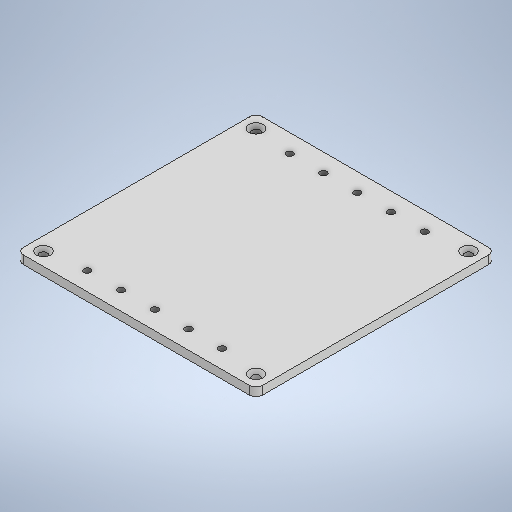
# Autodesk Inventor part: Chuck Adapter Plate
Saved by Autodesk Inventor 2025 (Build 290162000, 162)
## iProperties
Created: 2024-10-23
Part Number: Chuck Adapter Plate
Material: Generic
Document SubType Name: Modeling
Designer: Caleb Fangmeier
Density: 1 g/cm^3
Appearance: Default
Author: Caleb Fangmeier
Autodesk Inventor part; units mm, degrees
ref_plane "YZ Plane" through (0, 0, 0) normal (1, 0, 0) x (0, 1, 0)
ref_plane "XZ Plane" through (0, 0, 0) normal (0, 1, 0) x (-1, 0, 0)
ref_plane "XY Plane" through (0, 0, 0) normal (0, 0, 1) x (1, 0, 0)
sketch "Sketch1" plane through (0, 0, 0) normal (0, 1, 0) x (-1, 0, 0)
  line L0 (-90, -90) -> (90, -90)
  line L1 (90, -90) -> (90, 90)
  line L2 (90, 90) -> (-90, 90)
  line L3 (-90, 90) -> (-90, -90)
  line L4 (-90, -90) -> (90, 90) construction
  line L5 (90, -90) -> (-90, 90) construction
  point P0 (0, 0)
  dimension "d0" = 180
  dimension "d1" = 180
  constraints: 12 end point, 2 midpoint, 2 parallel, 1 horizontal, 1 perpendicular
  measures "d0" distance of L0.end L1.end
  measures "d1" distance of L1.end L2.end
extrude "Extrusion1" add sketch "Sketch1" along normal blind 6.35
sketch "Sketch2" plane through (0, 6.35, 0) normal (0, 1, 0) x (1, 0, 0)
  point P0 (0, 0)
  point P1 (-80, -80)
  point P2 (-80, 80)
  point P3 (80, 80)
  point P4 (80, -80)
  dimension "d4" = 160
  dimension "d5" = 80
  dimension "d6" = 160
  dimension "d7" = 80
  constraints: 2 horizontal alignment, 2 vertical alignment
  measures "d4" distance of point (-80, 80) point (-80, -80)
  measures "d5" horizontal distance of point (-80, -80) point (0, 0)
  measures "d6" distance of point (80, -80) point (-80, -80)
  measures "d7" horizontal distance of point (-80, -80) point (0, 0)
hole "Hole1" at (-80, 6.35, 80) at (-80, 6.35, -80) at (80, 6.35, -80) at (80, 6.35, 80) direction (0, -1, 0) diameter 5.5 end through all countersink diameter 10.4 countersink angle 90 clearance for "Flat Head Machine Screw" size "M5" standard "Ansi Metric M Profile"
sketch "Sketch3" plane through (0, 6.35, 0) normal (0, 1, 0) x (1, 0, 0)
  point P0 (0, 0)
  point P1 (-25.4, 76.2)
  point P2 (-25.4, -76.2)
  point P3 (25.4, -76.2)
  point P4 (25.4, 76.2)
  point P5 (0, -76.2)
  point P6 (0, 76.2)
  point P7 (-50.8, 76.2)
  point P8 (-50.8, -76.2)
  point P9 (50.8, -76.2)
  point P10 (50.8, 76.2)
  dimension "d15" = 152.4
  dimension "d16" = 50.8
  dimension "d17" = 76.2
  dimension "d18" = 25.4
  dimension "d27" = 25.4
  dimension "d28" = 25.4
  constraints: 8 horizontal alignment, 6 vertical alignment
  measures "d15" distance of point (-25.4, 76.2) point (-25.4, -76.2)
  measures "d16" distance of point (-25.4, -76.2) point (25.4, -76.2)
  measures "d17" vertical distance of point (-25.4, -76.2) point (0, 0)
  measures "d18" horizontal distance of point (-25.4, -76.2) point (0, 0)
  measures "d27" distance of point (50.8, -76.2) point (25.4, -76.2)
  measures "d28" distance of point (-50.8, -76.2) point (-25.4, -76.2)
hole "Hole2" at (-25.4, 6.35, -76.2) at (-25.4, 6.35, 76.2) at (25.4, 6.35, 76.2) at (25.4, 6.35, -76.2) at (0, 6.35, 76.2) at (-50.8, 6.35, 76.2) at (50.8, 6.35, 76.2) at (50.8, 6.35, -76.2) at (0, 6.35, -76.2) at (-50.8, 6.35, -76.2) direction (0, -1, 0) diameter 4.9784 end through all thread size "1/4-20 UNC" class "2B" standard "ANSI Unified Screw Threads"
fillet "Fillet1" radius 5 4 edges at (90, 3.175, 90) (90, 3.175, -90) (-90, 3.175, -90) (-90, 3.175, 90)
equation "\"d5\" = 0.5 * d4"
equation "\"d7\" = 0.5 * d6"
equation "\"d17\" = 0.5 * d15"
equation "\"d18\" = 0.5 * d16"
body "Solid1"
